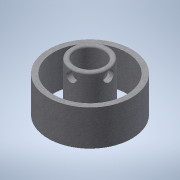
# Autodesk Inventor part: 2
Saved by Autodesk Inventor 2021 (Build 250183000, 183)
## iProperties
Created: 2012-06-12
Part Number: 2
Material: Genérico
Document SubType Name: Modeling
Designer: Luis
Density: 1 g/cm^3
Appearance: Inoxidable - Bruñido
Author: Luis
Autodesk Inventor part; units mm, degrees
ref_plane "YZ Plane" through (0, 0, 0) normal (1, 0, 0) x (0, 1, 0)
ref_plane "XZ Plane" through (0, 0, 0) normal (0, 1, 0) x (-1, 0, 0)
ref_plane "XY Plane" through (0, 0, 0) normal (0, 0, 1) x (1, 0, 0)
sketch "Sketch1" plane through (0, 0, 0) normal (0, 0, 1) x (1, 0, 0)
  circle A0 centre (0, 0) radius 24
  circle A1 centre (0, 0) radius 21
  circle A2 centre (0, 0) radius 8
  circle A3 centre (0, 0) radius 11
  dimension "d0" = 48
  dimension "d1" = 3
  dimension "d2" = 16
  dimension "d3" = 3
  constraints: 4 centre point, 4 coincident
  measures "d0" diameter of A0
  measures "d1" radial gap between concentric circles of A0 A1
  measures "d2" diameter of A2
  measures "d3" radial gap between concentric circles of A3 A2
extrude "Extrusion1" add sketch "Sketch1" along normal blind 20.5 contours A0
extrude "Extrusion2" add sketch "Sketch1" along normal blind 28.5 and the other way blind 4 contours A3
sketch "Sketch2" plane through (0, 0, 0) normal (0, 1, 0) x (-1, 0, 0)
  line L0 (-11, -4) -> (-11, 28.5) projected
  line L1 (-8, 28.5) -> (8, 28.5) projected
  line L2 (0, 28.5) -> (0, 24.5)
  circle A0 centre (0, 24.5) radius 3
  point P0 (0, 0)
  dimension "d10" = 4
  dimension "d11" = 6
  constraints: 2 end point, 1 centre point, 1 coincident, 1 midpoint, 1 perpendicular
  measures "d10" distance of L2.start L2.end
  measures "d11" diameter of A0
extrude "Extrusion3" cut sketch "Sketch2" against normal blind 28.5
sketch "Sketch3" plane through (0, 0, 0) normal (1, 0, 0) x (0, 1, 0)
  line L0 (-8, 28.5) -> (8, 28.5) projected
  line L1 (0, 28.5) -> (0, 24.5)
  circle A0 centre (0, 24.5) radius 3
  point P0 (0, 0)
  dimension "d14" = 4
  dimension "d15" = 6
  constraints: 2 end point, 1 centre point, 1 coincident, 1 midpoint, 1 perpendicular
  measures "d14" distance of L1.start L1.end
  measures "d15" diameter of A0
extrude "Extrusion4" cut sketch "Sketch3" along normal blind 28.5
fillet "Fillet1" radius 1 4 edges at (-11, 0, 28.5) (-8, 0, 28.5) (-11, 0, -4) (-8, 0, -4)
body "Solid1"
